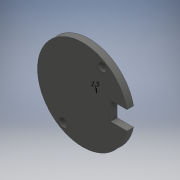
# Autodesk Inventor part: led_with_pad
Saved by Autodesk Inventor 2017 (Build 210142000, 142)
## iProperties
Created: 2018-04-05
Part Number: led_with_pad
Material: Generic
Document SubType Name: Modeling
Designer: dasae
Density: 1 g/cm^3
Appearance: Default
Author: dasae
Autodesk Inventor part; units mm, degrees
ref_plane "YZ Plane" through (0, 0, 0) normal (1, 0, 0) x (0, 1, 0)
ref_plane "XZ Plane" through (0, 0, 0) normal (0, 1, 0) x (-1, 0, 0)
sketch "Sketch1" plane through (0, 0, 0) normal (0, 1, 0) x (-1, 0, 0)
  arc A0 (-10.7674, -2.25) -> (-10.7674, 2.25) centre (0, 0) ccw
  circle A1 centre (0, 0) radius 9.5 construction
  line L0 (-10.7674, -2.25) -> (-6.7674, -2.25)
  line L1 (-6.7674, -2.25) -> (-6.7674, 2.25)
  line L2 (-6.7674, 2.25) -> (-10.7674, 2.25)
  arc A2 (0, -9.5) -> (8.2272, 4.75) centre (0, 0) ccw
  line L3 (0, 0) -> (0, -9.5) construction
  circle A3 centre (4.75, -8.2272) radius 1
  circle A4 centre (-4.7508, 8.2268) radius 1
  arc A5 (4.75, -8.2272) -> (9.5, 0) centre (0, 0) ccw
  line L4 (0, 0) -> (4.75, -8.2272) construction
  line L5 (0, 0) -> (9.5, 0) construction
  line L6 (4.75, -8.2272) -> (-4.7508, 8.2268)
  point P0 (8.2272, -4.75)
  dimension "d1" = 19
  dimension "d7" = 2
  dimension "d8" = 2
  dimension "d20" = 60
  constraints: 14 end point, 12 point on circle, 6 centre point, 6 coincident, 1 parallel
  measures "d1" diameter of A1
  measures "d7" diameter of A3
  measures "d8" diameter of A4
  measures "d20" angle of L4 L5
extrude "Extrusion1" add sketch "Sketch1" along normal blind 1.6
sketch "Sketch2" plane through (0, 1.6, 0) normal (0, 1, 0) x (1, 0, 0)
  circle A0 centre (0, 0) radius 1.25 construction
  line L0 (1.4943, -3.4321) -> (1.4943, 1.7978)
  line L1 (1.4943, 1.7978) -> (-1.4943, 1.7978)
  line L2 (-1.4943, 1.7978) -> (-1.4943, -3.4321)
  line L3 (-1.4943, -3.4321) -> (1.4943, -3.4321)
  line L4 (1.4943, -3.4321) -> (-1.4943, 1.7978) construction
  line L5 (1.4943, 1.7978) -> (-1.4943, -3.4321) construction
  point P0 (0, -0.8172)
  dimension "d11" = 2.5
  constraints: 12 end point, 2 midpoint, 2 parallel, 1 centre point, 1 coincident, 1 perpendicular, 1 vertical
  measures "d11" diameter of A0
extrude "Extrusion2" add sketch "Sketch2" along normal blind 1.6
sketch "Sketch3" plane through (0, 3.2, 0) normal (0, 1, 0) x (1, 0, 0)
  circle A0 centre (0, 0) radius 1.25
  line L0 (0, -1.25) -> (0, 1.25)
  dimension "d14" = 2.5
  constraints: 2 end point, 2 point on circle, 1 centre point, 1 coincident, 1 vertical
  measures "d14" diameter of A0
ref_plane "Work Plane1" through (0, 3.2, 1.25) normal (1, 0, 0) x (0, 0, -1)
sketch "Sketch4" plane through (0, 3.2, 1.25) normal (1, 0, 0) x (0, 0, -1)
  line L0 (-2.1821, 0) -> (3.0478, 0) projected
  line L1 (1.25, 0) -> (1.25, 0.5805)
  arc A0 (2.5038, 0) -> (1.25, 0.5805) centre (1.2852, -0.9877) ccw
  point P0 (1.25, -3.2)
  constraints: 2 end point, 2 point on circle, 2 point on line, 1 centre point, 1 vertical
revolve "Revolution1" add sketch "Sketch4" angle 360 about axis through (0, 3.2, 0) along (0, 1, 0)
sketch "Sketch5" plane through (0, 1.6, 0) normal (0, 1, 0) x (1, 0, 0)
  line L0 (-0.9227, 9.0998) -> (2.0026, 9.0998)
  line L1 (2.0026, 9.0998) -> (2.0026, 5.8604)
  line L2 (2.0026, 5.8604) -> (-0.9227, 5.8604)
  line L3 (-0.9227, 5.8604) -> (-0.9227, 9.0998)
  point P0 (0, 0)
  constraints: 8 end point, 2 parallel, 1 horizontal, 1 perpendicular
extrude "Extrusion3" add sketch "Sketch5" along normal blind 1.6
sketch "Sketch6" plane through (0, 1.6, 0) normal (0, 1, 0) x (1, 0, 0)
  point P0 (0, 0)
sketch "Sketch7" plane through (0, 1.6, 0) normal (0, 1, 0) x (1, 0, 0)
  line L0 (7.0213, -6.5083) -> (8.72, -5.0751)
  line L1 (8.72, -5.0751) -> (7.5239, -3.6574)
  line L2 (7.5239, -3.6574) -> (5.8251, -5.0906)
  line L3 (5.8251, -5.0906) -> (7.0213, -6.5083)
  line L4 (5.0154, -4.9785) -> (6.7141, -3.5452)
  line L5 (6.7141, -3.5452) -> (5.5179, -2.1275)
  line L6 (5.5179, -2.1275) -> (3.8192, -3.5608)
  line L7 (3.8192, -3.5608) -> (5.0154, -4.9785)
  line L8 (9.953, 0) -> (3.3605, 0) construction
  line L9 (7.0213, 6.5083) -> (8.72, 5.0751)
  line L10 (8.72, 5.0751) -> (7.5239, 3.6574)
  line L11 (7.5239, 3.6574) -> (5.8251, 5.0906)
  line L12 (5.8251, 5.0906) -> (7.0213, 6.5083)
  line L13 (5.0154, 4.9785) -> (6.7141, 3.5452)
  line L14 (6.7141, 3.5452) -> (5.5179, 2.1275)
  line L15 (5.5179, 2.1275) -> (3.8192, 3.5608)
  line L16 (3.8192, 3.5608) -> (5.0154, 4.9785)
  point P0 (0, 0)
  point P1 (8.2726, -4.0828)
  point P2 (8.2726, 4.0828)
  constraints: 34 end point, 9 symmetric about line, 4 parallel, 2 perpendicular, 1 horizontal
extrude "Extrusion4" add sketch "Sketch7" along normal blind 0.2
body "Solid1"
